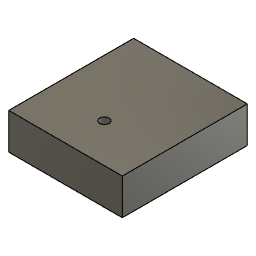
YBeltClampBracket v25 (Autodesk Fusion 360 archive; units mm, degrees)
design "YBeltClampBracket" references "tormach 770mx"
Autodesk Fusion 360 part; units mm, degrees
sketch "Sketch1" plane through (0, 0, 0) normal (0, 1, 0) x (1, 0, 0)
  line L0 (0, 0) -> (40, 0)
  line L1 (40, 0) -> (40, -44)
  line L2 (40, -44) -> (0, -44)
  line L3 (0, -44) -> (0, 0)
  dimension "d1" = 40
  dimension "d2" = 44
  constraint horizontal L0
  constraint vertical L1
  constraint horizontal L2
  constraint vertical L3
  constraint coincident L0.start L3.end
  measures "d1" distance of L0.start L0.end
  measures "d2" distance of L0.start L2.end
extrude "Extrude1" add sketch "Sketch1" along normal blind 12.7
sketch "Sketch2" plane through (0, 12.7, 0) normal (0, 1, 0) x (-1, 0, 0)
  line L0 (0, 44) -> (-40, 44)
  line L1 (-40, 44) -> (-40, 0)
  line L2 (-40, 0) -> (0, 0)
  line L3 (0, 0) -> (0, 44)
  line L4 (0, 30.3) -> (-40, 30.3) construction
  point P0 (-20, 30.3)
  dimension "d38" = 30.3
  constraint midpoint L4 P0
  measures "d38" distance of L2 L4
hole "Hole8" at (20, 12.7, 30.3) direction (0, -1, 0) diameter 3.3 end through all
sketch "Sketch4" plane through (0, 0, 0) normal (0, 0, -1) x (-1, 0, 0)
  line L0 (-40, 0) -> (0, 0)
  line L1 (0, 0) -> (0, 12.7)
  line L2 (0, 12.7) -> (-40, 12.7)
  line L3 (-40, 12.7) -> (-40, 0)
  line L4 (-40, 7.7) -> (0, 7.7) construction
  line L5 (-20, 12.7) -> (-20, 0) construction
  point P0 (-35, 7.7)
  point P1 (-5, 7.7)
  point P2 (-20, 7.7)
  dimension "d39" = 5
  dimension "d40" = 15
  dimension "d41" = 15
  constraint coincident L3 L4.start
  constraint coincident L1 L4.end
  constraint perpendicular L1 L4
  constraint midpoint L2 L5.start
  constraint midpoint L0 L5.end
  constraint coincident L4 P0
  constraint coincident L4 P1
  constraint midpoint L4 P2
  measures "d39" distance of L2 L4
  measures "d40" distance of L5 P0
  measures "d41" distance of L5 P1
hole "Hole9" at (35, 7.7, 0) direction (0, 0, 1) diameter 4.3 depth 10 tip angle 118
hole "Hole10" at (5, 7.7, 0) direction (0, 0, 1) diameter 4.3 depth 10 tip angle 118
hole "Hole11" at (20, 7.7, 0) direction (0, 0, 1) diameter 4.3 depth 10 tip angle 118
